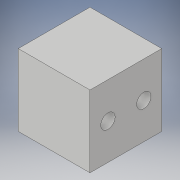
# Autodesk Inventor part: cube fixation2
Saved by Autodesk Inventor 2017 (Build 210142000, 142)
## iProperties
Created: 2018-11-10
Part Number: cube fixation2
Material: Generic
Document SubType Name: Modeling
Designer: Antoine Blaud
Density: 1 g/cm^3
Appearance: Default
Author: Antoine Blaud
Autodesk Inventor part; units mm, degrees
ref_plane "YZ Plane" through (0, 0, 0) normal (1, 0, 0) x (0, 1, 0)
ref_plane "XZ Plane" through (0, 0, 0) normal (0, 1, 0) x (-1, 0, 0)
ref_plane "XY Plane" through (0, 0, 0) normal (0, 0, 1) x (1, 0, 0)
sketch "Sketch1" plane through (0, 0, 0) normal (1, 0, 0) x (0, 1, 0)
  line L0 (-19.05, 19.05) -> (19.05, 19.05)
  line L1 (19.05, 19.05) -> (19.05, -19.05)
  line L2 (19.05, -19.05) -> (-19.05, -19.05)
  line L3 (-19.05, -19.05) -> (-19.05, 19.05)
  line L4 (-19.05, 19.05) -> (19.05, -19.05) construction
  line L5 (19.05, 19.05) -> (-19.05, -19.05) construction
  line L6 (19.05, 19.05) -> (-19.05, -19.05)
  line L7 (19.05, -19.05) -> (-19.05, 19.05)
  line L8 (0, 0) -> (0, -19.05)
  line L9 (0, 0) -> (0, 19.05)
  circle A0 centre (0, 9.525) radius 3.81
  circle A1 centre (0, -9.525) radius 3.81
  dimension "d0" = 38.1
  dimension "d1" = 38.1
  dimension "d2" = 7.62
  dimension "d3" = 7.62
  dimension "d4" = 19.05
  constraints: 20 end point, 6 midpoint, 2 centre point, 2 coincident, 2 parallel, 1 horizontal, 1 perpendicular
  measures "d0" distance of L1.end L2.end
  measures "d1" distance of L0.end L1.end
  measures "d2" diameter of A0
  measures "d3" diameter of A1
  measures "d4" distance of point (0, -9.525) A0.centre
extrude "Extrusion1" add sketch "Sketch1" along normal blind 38.1 contours L7 L6 L3 | L0 L9 A0 L7 | L0 L6 L9 A0 | L6 L8 A1 L2 | L6 L1 L7 | L7 L2 L8 A1
sketch "Sketch2" plane through (0, -19.05, -19.05) normal (0, -1, 0) x (1, 0, 0)
  line L0 (38.1, 0) -> (38.1, 38.1) projected
  line L1 (0, 0) -> (38.1, 0) projected
  line L2 (38.1, 38.1) -> (38.1, 0)
  line L3 (38.1, 0) -> (0, 0)
  line L4 (0, 0) -> (0, 38.1) projected
  line L5 (0, 0) -> (0, 38.1)
  line L6 (0, 38.1) -> (38.1, 38.1)
  line L7 (0, 38.1) -> (38.1, 38.1) projected
  line L8 (0, 0) -> (38.1, 38.1)
  line L9 (38.1, 0) -> (0, 38.1)
  circle A0 centre (19.05, 19.05) radius 12.5
  point P0 (0, 19.05)
  dimension "d7" = 25
  constraints: 12 end point, 2 collinear, 2 perpendicular, 1 centre point, 1 midpoint
  measures "d7" diameter of A0
extrude "Extrusion2" cut sketch "Sketch2" against normal blind 15 contours A0 L8 L9 | L9 L8 A0 | L8 L9 A0 | A0 L9 L8
body "Solid1"
